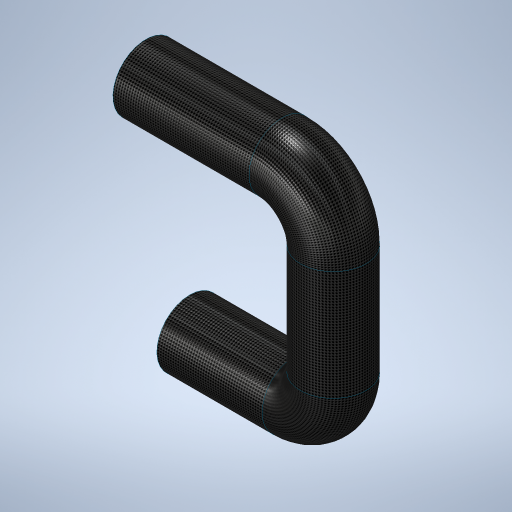
# Autodesk Inventor part: vacuum
Saved by Autodesk Inventor 2024 (Build 280153000, 153)
## iProperties
Created: 2023-07-07
Part Number: vacuum
Material: Generic
Document SubType Name: Modeling
Designer: gaura
Density: 1 g/cm^3
Appearance: Sky Blue Medium
Author: gaura
Autodesk Inventor part; units mm, degrees
ref_plane "YZ Plane" through (0, 0, 0) normal (1, 0, 0) x (0, 1, 0)
ref_plane "XZ Plane" through (0, 0, 0) normal (0, 1, 0) x (-1, 0, 0)
ref_plane "XY Plane" through (0, 0, 0) normal (0, 0, 1) x (1, 0, 0)
sketch "Sketch1" plane through (0, 0, 0) normal (1, 0, 0) x (0, 1, 0)
  circle A0 centre (-37.5, 0) radius 37.5
  point P0 (0, 0)
  dimension "d7" = 75
  constraints: 1 centre point
  measures "d7" diameter of A0
sketch3d "3D Sketch2"
  line L0 (0, -24, 0) -> (120, -24, 0)
  arc A0 (120, -24, 0) -> (150, 6, 0) centre (120, 6, 0) ccw
  line L1 (150, 6, 0) -> (150, 131, 0)
  arc A1 (150, 131, 0) -> (105, 176, 0) centre (105, 131, 0) ccw
  line L2 (105, 176, 0) -> (-50, 176, 0)
  dimension "d0" = 150
  dimension "d1" = 200
  dimension "d2" = 30
  dimension "d3" = 200
  dimension "d4" = 45
sweep "Sweep1" add profiles "Sketch1" path "3D Sketch2"
sketch "Sketch2" plane through (-50, 189.5, 0) normal (-1, 0, 0) x (0, 0, 1)
  circle A0 centre (0, 0) radius 30
  point P0 (0, -189.5)
  dimension "d10" = 60
  constraints: 1 centre point
  measures "d10" diameter of A0
extrude "Extrusion1" cut sketch "Sketch2" against normal blind 170
sketch "Sketch3" plane through (0, -37.5, 0) normal (-1, 0, 0) x (0, 0, 1)
  circle A0 centre (0, 0) radius 30
  point P0 (0, 37.5)
  dimension "d13" = 60
  constraints: 1 centre point
  measures "d13" diameter of A0
extrude "Extrusion2" cut sketch "Sketch3" against normal blind 150
body "Solid1"
